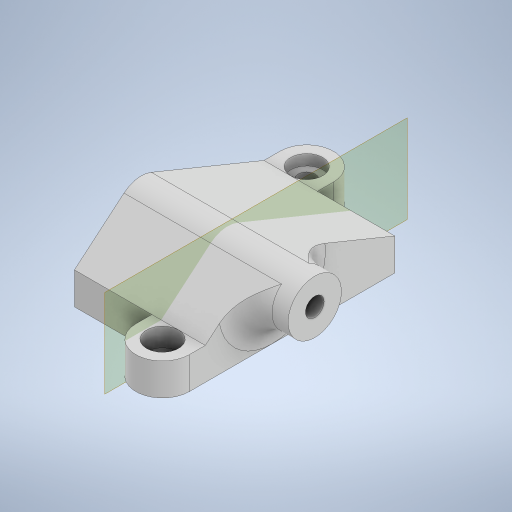
# Autodesk Inventor part: uchwyt_gorny
Saved by Autodesk Inventor 2023 (Build 270158000, 158)
## iProperties
Created: 2024-05-12
Part Number: uchwyt_gorny
Material: Ogólny
Document SubType Name: Modeling
Designer: kamil
Density: 1 g/cm^3
Appearance: Domyślna
Author: kamil
Autodesk Inventor part; units mm, degrees
ref_plane "YZ Plane" through (0, 0, 0) normal (1, 0, 0) x (0, 1, 0)
ref_plane "XZ Plane" through (0, 0, 0) normal (0, 1, 0) x (-1, 0, 0)
ref_plane "XY Plane" through (0, 0, 0) normal (0, 0, 1) x (1, 0, 0)
sketch "Szkic1" plane through (0, 0, 0) normal (0, 1, 0) x (-1, 0, 0)
  circle A0 centre (-29, 62.25) radius 3
  circle A1 centre (-14.5, 20.75) radius 3
  line L0 (5, -17.75) -> (5, 17.75)
  line L1 (5, 17.75) -> (4.2, 17.75)
  line L2 (-9.5, 20.75) -> (-9.5, 17.75)
  arc A2 (-9.5, 20.75) -> (-19.5, 20.75) centre (-14.5, 20.75) ccw
  line L3 (-19.5, 17.75) -> (-19.5, 20.75)
  line L4 (-19.5, -17.75) -> (-19.5, 17.75)
  line L5 (-16.25, -17.75) -> (-19.5, -17.75)
  line L6 (-5, -20.75) -> (-5, -17.75)
  arc A3 (-5, -20.75) -> (5, -20.75) centre (0, -20.75) ccw
  line L7 (5, -17.75) -> (5, -20.75)
  circle A4 centre (-14.5, 20.75) radius 3 projected
  circle A5 centre (0, -20.75) radius 1.6 projected
  line L8 (-5, -17.75) -> (-16.25, -17.75)
  line L9 (-9.5, 17.75) -> (4.2, 17.75)
  point P0 (0, 0)
  point P1 (0, 0)
  constraints: 20 end point, 4 centre point, 4 point on circle, 1 collinear, 1 horizontal
extrude "Wyciągnięcie proste1" add sketch "Szkic1" along normal blind 6 contours L7 A3 L6 L8 L5 L4 L3 A2 L2 L9 L1 L0 | A5
sketch "Szkic2" plane through (0, 0, 0) normal (0, -1, 0) x (1, 0, 0)
  circle A0 centre (14.5, 20.75) radius 3 projected
  circle A1 centre (0, -20.75) radius 3 projected
  circle A2 centre (0, -20.75) radius 1.6
  circle A3 centre (14.5, 20.75) radius 1.6
  point P0 (0, 0)
  dimension "d3" = 3.2
  dimension "d4" = 3.2
  constraints: 2 centre point, 2 coincident
  measures "d3" diameter of A2
  measures "d4" diameter of A3
extrude "Wyciągnięcie proste2" add sketch "Szkic2" against normal blind 2.5
sketch "Szkic3" plane through (-5, 0, -17.75) normal (-1, 0, 0) x (0, 0, 1)
  line L0 (0, 0) -> (0, 6)
  line L1 (35.5, 0) -> (35.5, 6)
  line L2 (35.5, 0) -> (0, 0) construction
  line L3 (23, 0) -> (23, 10) construction
  circle A0 centre (23, 10) radius 5
  line L4 (0, 6) -> (21.108128, 14.628263)
  line L5 (35.5, 6) -> (26.223183, 13.822446)
  line L6 (-3, 6) -> (35.5, 6)
  point P0 (17.75, 0)
  dimension "d7" = 12.5
  dimension "d8" = 10
  dimension "d9" = 10
  constraints: 6 end point, 2 coincident, 2 point on circle, 2 tangent, 1 centre point, 1 point on line, 1 vertical
  measures "d7" distance between parallel lines of L1 L3
  measures "d8" distance of L3.start L3.end
  measures "d9" diameter of A0
extrude "Wyciągnięcie proste3" add sketch "Szkic3" against normal up to surface (24.5 mm away) contours A0 L6 | A0 L5 L6 | A0 L6 L4 picked at (21.41132, 10.424905)
sketch "Szkic4" plane through (-5, 0, -17.75) normal (-1, 0, 0) x (0, 0, 1)
  line L0 (-3, 0) -> (35.5, 0)
  line L1 (35.5, 0) -> (35.5, 6)
  line L2 (-3, 6) -> (0, 6)
  line L3 (-3, 0) -> (-3, 6)
  line L4 (35.5, 6) -> (26.223183, 13.822446)
  arc A0 (26.223183, 13.822446) -> (21.108128, 14.628263) centre (23, 10) ccw
  line L5 (21.108128, 14.628263) -> (0, 6)
  point P0 (17.75, 0)
hole "Otwór1" at (-5, 10, 5.25) direction (1, 0, 0) diameter 3.5 end through all
sketch "Szkic5" plane through (0, 6, 0) normal (0, 1, 0) x (1, 0, 0)
  arc A0 (5, 20.75) -> (-5, 20.75) centre (0, 20.75) ccw projected
  point P0 (0, 0)
hole "Otwór2" at (0, 6, -20.75) direction (0, -1, 0) diameter 3.2 end through all counterbore diameter 6 counterbore depth 2
sketch "Szkic6" plane through (19.5, 0, 20.75) normal (1, 0, 0) x (0, 0, -1)
  circle A0 centre (15.5, 10) radius 1.75
  line L0 (0, 0) -> (38.5, 0)
  line L1 (38.5, 0) -> (38.5, 6)
  line L2 (17.391872, 14.628263) -> (38.5, 6)
  arc A1 (17.391872, 14.628263) -> (12.276817, 13.822446) centre (15.5, 10) ccw
  line L3 (3, 6) -> (12.276817, 13.822446)
  line L4 (0, 6) -> (3, 6)
  line L5 (0, 0) -> (0, 6)
  circle A2 centre (15.5, 10) radius 5
  point P0 (20.75, 0)
  point P1 (12.276817, 13.822446)
  point P2 (17.391872, 14.628263)
  constraints: 1 centre point, 1 coincident
extrude "Wyciągnięcie proste4" add sketch "Szkic6" along normal blind 8 contours A2 A1
fillet "Zaokrąglenie1" radius 5 1 edges at (19.5, 5.0609, 4.4719)
ref_plane "Płaszczyzna konstrukcyjna1" through (11.25, 0, -20.75) normal (-1, 0, 0) x (0, 0, 1)
sketch "Szkic7" plane through (11.25, 0, -20.75) normal (-1, 0, 0) x (0, 0, 1)
  circle A0 centre (26, 10) radius 1.75
  circle A1 centre (26, 10) radius 3.25
  line L0 (26, 10) -> (26, 0)
  line L1 (0, 0) -> (38.5, 0)
  line L2 (32, 0) -> (29.142437, 10.829212)
  line L3 (22.857563, 10.829212) -> (20, 0)
  point P0 (20.75, 0)
  dimension "d29" = 6.5
  dimension "d30" = 6
  dimension "d31" = 6
  constraints: 6 end point, 3 point on line, 2 point on circle, 2 tangent, 1 centre point, 1 coincident, 1 vertical
  measures "d29" diameter of A1
  measures "d30" distance of L0.end L2.start
  measures "d31" distance of L0.end L3.end
extrude "Wyciągnięcie proste5" cut sketch "Szkic7" along normal blind 10 and the other way blind 1 contours A0 | A1 | A1 L2 L1 L0 | L0 L1 L3 A1
sketch "Szkic8" plane through (11.25, 0, -20.75) normal (-1, 0, 0) x (0, 0, 1)
  circle A0 centre (26, 10) radius 1.75
  circle A1 centre (26, 10) radius 2.9
  line L0 (28.9, 8.325684) -> (26, 6.651368)
  line L1 (26, 6.651368) -> (23.1, 8.325684)
  line L2 (23.1, 8.325684) -> (23.1, 11.674316)
  line L3 (23.1, 11.674316) -> (26, 13.348632)
  line L4 (26, 13.348632) -> (28.9, 11.674316)
  line L5 (28.9, 11.674316) -> (28.9, 8.325684)
  point P0 (20.75, 0)
  point P1 (28.9, 10)
  dimension "d36" = 5.8
  constraints: 12 end point, 2 coincident, 1 horizontal alignment, 1 midpoint, 15 other
extrude "Wyciągnięcie proste6" cut sketch "Szkic8" along normal blind 13 and the other way blind 3 contours A0 | A1 | L5 L0 A1 | A1 L4 L5 | A1 L3 L4 | L0 L1 A1 | A1 L2 L3 | L1 L2 A1
